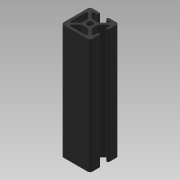
# Autodesk Inventor part: 25-2502-BLACK-FB
Saved by Autodesk Inventor 2013 (Build 170138000, 138)
## iProperties
Company: 80/20 Inc.
Created: 2014-04-23
Part Number: 25-2502-BLACK-FB
Material: Generic
Document SubType Name: Modeling
Designer: Ross Bowman
Density: 1 g/cm^3
Engineer: Ross Bowman
Catalog Web Link: 8020.net
Vendor: 80/20 Inc.
Material: 6105-T5 Aluminum
Author: Ross Bowman
Keywords: 80/20 , 8020 , T-Slot , Extrusion
Autodesk Inventor part; units mm, degrees
ref_plane "YZ Plane" through (0, 0, 0) normal (1, 0, 0) x (0, 1, 0)
ref_plane "XZ Plane" through (0, 0, 0) normal (0, 1, 0) x (-1, 0, 0)
ref_plane "XY Plane" through (0, 0, 0) normal (0, 0, 1) x (1, 0, 0)
sketch "Sketch1" plane through (0, 0, 0) normal (0, 0, 1) x (1, 0, 0)
  arc A0 (-10.36, -6.4282) -> (-8.6498, -7.1366) centre (-9.3582, -6.4282) ccw
  line L0 (-10.36, 6.4282) -> (-10.36, -6.4282)
  arc A1 (-8.6498, 7.1366) -> (-10.36, 6.4282) centre (-9.3582, 6.4282) ccw
  line L1 (-5.1567, 3.6435) -> (-8.6498, 7.1366)
  arc A2 (-4.38, 1.7684) -> (-5.1567, 3.6435) centre (-7.0317, 1.7684) ccw
  line L2 (-4.38, -1.7684) -> (-4.38, 1.7684)
  arc A3 (-5.1567, -3.6435) -> (-4.38, -1.7684) centre (-7.0317, -1.7684) ccw
  line L3 (-8.6498, -7.1366) -> (-5.1567, -3.6435)
  arc A4 (-1.7684, -4.38) -> (-3.6435, -5.1567) centre (-1.7684, -7.0317) ccw
  line L4 (1.7684, -4.38) -> (-1.7684, -4.38)
  arc A5 (3.6435, -5.1567) -> (1.7684, -4.38) centre (1.7684, -7.0317) ccw
  line L5 (7.1366, -8.6498) -> (3.6435, -5.1567)
  arc A6 (6.4282, -10.36) -> (7.1366, -8.6498) centre (6.4282, -9.3582) ccw
  line L6 (-6.4282, -10.36) -> (6.4282, -10.36)
  arc A7 (-7.1366, -8.6498) -> (-6.4282, -10.36) centre (-6.4282, -9.3582) ccw
  line L7 (-3.6435, -5.1567) -> (-7.1366, -8.6498)
  circle A8 centre (0, 0) radius 2.5
  arc A9 (-4.32, 10.36) -> (-4.32, 12.5) centre (-4.32, 11.43) ccw
  line L8 (-4.32, 12.5) -> (-10.5183, 12.5)
  arc A10 (-10.5183, 12.5) -> (-12.5, 10.5183) centre (-10.5183, 10.5183) ccw
  line L9 (-12.5, 10.5183) -> (-12.5, -10.5183)
  arc A11 (-12.5, -10.5183) -> (-10.5183, -12.5) centre (-10.5183, -10.5183) ccw
  line L10 (-10.5183, -12.5) -> (10.5183, -12.5)
  arc A12 (10.5183, -12.5) -> (12.5, -10.5183) centre (10.5183, -10.5183) ccw
  line L11 (12.5, -10.5183) -> (12.5, -4.32)
  arc A13 (12.5, -4.32) -> (10.36, -4.32) centre (11.43, -4.32) ccw
  line L12 (10.36, -4.32) -> (10.36, -6.4282)
  arc A14 (8.6498, -7.1366) -> (10.36, -6.4282) centre (9.3582, -6.4282) ccw
  line L13 (8.6498, -7.1366) -> (5.1567, -3.6435)
  arc A15 (4.38, -1.7684) -> (5.1567, -3.6435) centre (7.0317, -1.7684) ccw
  line L14 (4.38, -1.7684) -> (4.38, 1.7684)
  arc A16 (5.1567, 3.6435) -> (4.38, 1.7684) centre (7.0317, 1.7684) ccw
  line L15 (5.1567, 3.6435) -> (8.6498, 7.1366)
  arc A17 (10.36, 6.4282) -> (8.6498, 7.1366) centre (9.3582, 6.4282) ccw
  line L16 (10.36, 6.4282) -> (10.36, 4.32)
  arc A18 (10.36, 4.32) -> (12.5, 4.32) centre (11.43, 4.32) ccw
  line L17 (12.5, 4.32) -> (12.5, 10.5183)
  arc A19 (12.5, 10.5183) -> (10.5183, 12.5) centre (10.5183, 10.5183) ccw
  line L18 (10.5183, 12.5) -> (4.32, 12.5)
  arc A20 (4.32, 12.5) -> (4.32, 10.36) centre (4.32, 11.43) ccw
  line L19 (4.32, 10.36) -> (6.4282, 10.36)
  arc A21 (7.1366, 8.6498) -> (6.4282, 10.36) centre (6.4282, 9.3582) ccw
  line L20 (7.1366, 8.6498) -> (3.6435, 5.1567)
  arc A22 (1.7684, 4.38) -> (3.6435, 5.1567) centre (1.7684, 7.0317) ccw
  line L21 (1.7684, 4.38) -> (-1.7684, 4.38)
  arc A23 (-3.6435, 5.1567) -> (-1.7684, 4.38) centre (-1.7684, 7.0317) ccw
  line L22 (-3.6435, 5.1567) -> (-7.1366, 8.6498)
  arc A24 (-6.4282, 10.36) -> (-7.1366, 8.6498) centre (-6.4282, 9.3582) ccw
  line L23 (-6.4282, 10.36) -> (-4.32, 10.36)
  constraints: 48 end point, 48 point on circle, 25 centre point
extrude "Extrusion1" add sketch "Sketch1" against normal blind 100
body "Solid1"
